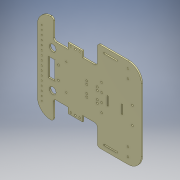
# Autodesk Inventor part: КВ33.035.002 - Платформа 3мм
Saved by Autodesk Inventor 2017 SP1 (Build 210196100, 196)
## iProperties
Part Number: КВ33.035.002 - Платформа 3мм
Material: Типовые
Document SubType Name: Modeling
Designer: sbnnl
Density: 1 g/cm^3
Appearance: Гладкий — пепельный
Author: sbnnl
Autodesk Inventor part; units mm, degrees
ref_plane "YZ Plane" through (0, 0, 0) normal (1, 0, 0) x (0, 1, 0)
ref_plane "XZ Plane" through (0, 0, 0) normal (0, 1, 0) x (-1, 0, 0)
ref_plane "XY Plane" through (0, 0, 0) normal (0, 0, 1) x (1, 0, 0)
sketch "Эскиз1" plane through (0, 0, 0) normal (0, 1, 0) x (-1, 0, 0)
  line L0 (0, 0) -> (93.3924, 0) construction
  line L1 (0, 72) -> (0, 0)
  line L2 (236.5, 0) -> (236.5, 72)
  line L3 (166.5, 57) -> (166.5, 70)
  line L4 (166.5, 70) -> (133.5, 70)
  line L5 (133.5, 70) -> (133.5, 57)
  line L6 (200, 57) -> (166.5, 57)
  line L7 (133.5, 57) -> (100, 57)
  line L8 (170.1825, 65) -> (127.9093, 65) construction
  circle A0 centre (150, 65) radius 2
  circle A1 centre (160, 65) radius 2
  circle A2 centre (140, 65) radius 2
  line L9 (150, 70) -> (150, 80.9563) construction
  line L10 (200, 57) -> (200, 102)
  line L11 (206.5, 102) -> (200, 102)
  line L12 (100, 57) -> (100, 102)
  line L13 (100, 102) -> (30, 102)
  arc A3 (236.5, 72) -> (206.5, 102) centre (206.5, 72) ccw
  arc A4 (30, 102) -> (0, 72) centre (30, 72) ccw
  line L14 (0, -72) -> (0, 0)
  line L15 (236.5, 0) -> (236.5, -72)
  line L16 (166.5, -70) -> (133.5, -70)
  line L17 (133.5, -70) -> (133.5, -57)
  line L18 (200, -57) -> (166.5, -57)
  line L19 (133.5, -57) -> (100, -57)
  line L20 (170.1825, -65) -> (127.9093, -65) construction
  circle A5 centre (150, -65) radius 2
  circle A6 centre (140, -65) radius 2
  line L21 (150, -70) -> (150, -80.9563) construction
  line L22 (200, -57) -> (200, -102)
  line L23 (206.5, -102) -> (200, -102)
  line L24 (100, -57) -> (100, -102)
  line L25 (100, -102) -> (30, -102)
  arc A7 (206.5, -102) -> (236.5, -72) centre (206.5, -72) ccw
  arc A8 (0, -72) -> (30, -102) centre (30, -72) ccw
  line L26 (166.5, -57) -> (166.5, -70)
  circle A9 centre (160, -65) radius 2
  dimension "d0" = 13
  dimension "d1" = 33
  dimension "d2" = 5
  dimension "d3" = 4
  dimension "d4" = 4
  dimension "d5" = 4
  dimension "d6" = 10
  dimension "d7" = 10
  dimension "d8" = 70
  dimension "d9" = 50
  dimension "d11" = 50
  dimension "d12" = 45
  dimension "d13" = 100
  dimension "d14" = 65
  dimension "d15" = 30
  constraints: 54 end point, 21 symmetric about line, 10 centre point, 10 point on line, 8 point on circle, 7 perpendicular, 4 horizontal, 4 tangent, 4 vertical, 2 collinear, 1 equal radius, 1 midpoint, 1 parallel, 5 other
  measures "d0" distance of L3.start L3.end
  measures "d1" distance of L3.end L4.end
  measures "d2" distance between parallel lines of L8 L4
  measures "d3" diameter of A0
  measures "d4" diameter of A1
  measures "d5" diameter of A2
  measures "d6" distance of A1.centre A0.centre
  measures "d7" distance of A2.centre A0.centre
  measures "d8" distance between parallel lines of L2 L3
  measures "d9" distance between parallel lines of L9 L10
  measures "d11" distance between parallel lines of L12 L9
  measures "d12" distance of L7.end L12.end
  measures "d13" distance between parallel lines of L12 L1
  measures "d14" distance between parallel lines of L0 L8
  measures "d15" radius of A3
extrude "Выдавливание1" add sketch "Эскиз1" along normal blind 3
sketch "Эскиз2" plane through (0, 3, 0) normal (0, 1, 0) x (1, 0, 0)
  line L0 (-20, -13.2915) -> (-20, 12.9921) construction
  circle A0 centre (-20, -20) radius 2
  circle A1 centre (-20, 20) radius 2
  point P0 (0, 0)
  dimension "d18" = 4
  dimension "d19" = 20
  dimension "d20" = 40
  dimension "d21" = 20
  constraints: 2 centre point, 2 end point, 2 point on line, 1 equal radius, 1 vertical
  measures "d18" diameter of A1
  measures "d19" distance from line of L0 point (0, 0)
  measures "d20" distance of A1.centre A0.centre
  measures "d21" horizontal distance of point (0, 0) A0.centre
extrude "Выдавливание2" cut sketch "Эскиз2" against normal blind 4
sketch "Эскиз3" plane through (0, 3, 0) normal (0, 1, 0) x (1, 0, 0)
  line L0 (-211.5, -21) -> (-196.5, -21)
  line L1 (-196.5, -21) -> (-196.5, 21)
  line L2 (-196.5, 21) -> (-211.5, 21)
  line L3 (-211.5, 21) -> (-211.5, -21)
  line L4 (-236.5, 72) -> (-236.5, -72) projected
  line L5 (-188.5, -21.5288) -> (-188.5, 22.9768) construction
  circle A0 centre (-188.5, -15) radius 2
  circle A1 centre (-188.5, 15) radius 2
  point P0 (0, 0)
  dimension "d24" = 42
  dimension "d25" = 15
  dimension "d26" = 40
  dimension "d27" = 21
  dimension "d28" = 4
  dimension "d29" = 4
  dimension "d31" = 6
  dimension "d32" = 8
  dimension "d33" = 30
  constraints: 10 end point, 2 centre point, 2 parallel, 2 point on line, 1 horizontal, 1 perpendicular, 1 vertical
  measures "d24" distance of L2.end L0.start
  measures "d25" distance of L1.end L2.end
  measures "d26" distance between parallel lines of L4 L1
  measures "d27" distance from line of point (0, 0) L2
  measures "d28" diameter of A0
  measures "d29" diameter of A1
  measures "d31" distance from line of A1.centre L2
  measures "d32" distance between parallel lines of L1 L5
  measures "d33" distance of A1.centre A0.centre
extrude "Выдавливание3" cut sketch "Эскиз3" against normal blind 4
sketch "Эскиз5" plane through (0, 3, 0) normal (0, 1, 0) x (1, 0, 0)
  line L0 (-134.2143, -16) -> (-95.4487, -16) construction
  circle A0 centre (-100, -16) radius 2
  line L1 (-100, -57) -> (-100, -102) projected
  line L2 (-100, -102) -> (-30, -102) projected
  line L3 (-236.5, -72) -> (-236.5, 72) projected
  line L4 (-236.5, 0) -> (-246.7698, 0) construction
  line L5 (-226.5, -8.1668) -> (-226.5, -72) construction
  circle A1 centre (-226.5, -5) radius 1.5
  circle A2 centre (-226.5, -15) radius 1.5
  circle A3 centre (-226.5, -25) radius 1.5
  circle A4 centre (-226.5, -35) radius 1.5
  circle A5 centre (-226.5, -45) radius 1.5
  circle A6 centre (-226.5, -55) radius 1.5
  circle A7 centre (-226.5, -65) radius 1.5
  circle A8 centre (-226.5, -75) radius 1.5
  circle A9 centre (-226.5, 5) radius 1.5
  circle A10 centre (-226.5, -5) radius 1.5
  circle A11 centre (-226.5, -15) radius 1.5
  circle A12 centre (-226.5, -25) radius 1.5
  circle A13 centre (-226.5, -35) radius 1.5
  circle A14 centre (-226.5, -45) radius 1.5
  circle A15 centre (-226.5, -55) radius 1.5
  circle A16 centre (-226.5, -65) radius 1.5
  circle A17 centre (-226.5, 15) radius 1.5
  circle A18 centre (-226.5, 5) radius 1.5
  circle A19 centre (-226.5, -5) radius 1.5
  circle A20 centre (-226.5, -15) radius 1.5
  circle A21 centre (-226.5, -25) radius 1.5
  circle A22 centre (-226.5, -35) radius 1.5
  circle A23 centre (-226.5, -45) radius 1.5
  circle A24 centre (-226.5, -55) radius 1.5
  circle A25 centre (-226.5, 25) radius 1.5
  circle A26 centre (-226.5, 15) radius 1.5
  circle A27 centre (-226.5, 5) radius 1.5
  circle A28 centre (-226.5, -5) radius 1.5
  circle A29 centre (-226.5, -15) radius 1.5
  circle A30 centre (-226.5, -25) radius 1.5
  circle A31 centre (-226.5, -35) radius 1.5
  circle A32 centre (-226.5, -45) radius 1.5
  circle A33 centre (-226.5, 35) radius 1.5
  circle A34 centre (-226.5, 25) radius 1.5
  circle A35 centre (-226.5, 15) radius 1.5
  circle A36 centre (-226.5, 5) radius 1.5
  circle A37 centre (-226.5, -5) radius 1.5
  circle A38 centre (-226.5, -15) radius 1.5
  circle A39 centre (-226.5, -25) radius 1.5
  circle A40 centre (-226.5, -35) radius 1.5
  circle A41 centre (-226.5, 45) radius 1.5
  circle A42 centre (-226.5, 35) radius 1.5
  circle A43 centre (-226.5, 25) radius 1.5
  circle A44 centre (-226.5, 15) radius 1.5
  circle A45 centre (-226.5, 5) radius 1.5
  circle A46 centre (-226.5, -5) radius 1.5
  circle A47 centre (-226.5, -15) radius 1.5
  circle A48 centre (-226.5, -25) radius 1.5
  circle A49 centre (-226.5, 55) radius 1.5
  circle A50 centre (-226.5, 45) radius 1.5
  circle A51 centre (-226.5, 35) radius 1.5
  circle A52 centre (-226.5, 25) radius 1.5
  circle A53 centre (-226.5, 15) radius 1.5
  circle A54 centre (-226.5, 5) radius 1.5
  circle A55 centre (-226.5, -5) radius 1.5
  circle A56 centre (-226.5, -15) radius 1.5
  circle A57 centre (-226.5, 65) radius 1.5
  circle A58 centre (-226.5, 55) radius 1.5
  circle A59 centre (-226.5, 45) radius 1.5
  circle A60 centre (-226.5, 35) radius 1.5
  circle A61 centre (-226.5, 25) radius 1.5
  circle A62 centre (-226.5, 15) radius 1.5
  circle A63 centre (-226.5, 5) radius 1.5
  circle A64 centre (-226.5, -5) radius 1.5
  circle A65 centre (-226.5, 75) radius 1.5
  circle A66 centre (-226.5, 65) radius 1.5
  circle A67 centre (-226.5, 55) radius 1.5
  circle A68 centre (-226.5, 45) radius 1.5
  circle A69 centre (-226.5, 35) radius 1.5
  circle A70 centre (-226.5, 25) radius 1.5
  circle A71 centre (-226.5, 15) radius 1.5
  circle A72 centre (-226.5, 5) radius 1.5
  line L6 (-78, -10) -> (-75, -10)
  line L7 (-75, -10) -> (-75, 10)
  line L8 (-75, 10) -> (-78, 10)
  line L9 (-78, 10) -> (-78, -10)
  line L10 (-133.5, -70) -> (-133.5, -57) projected
  line L11 (-45, -10) -> (-42, -10)
  line L12 (-42, -10) -> (-42, 10)
  line L13 (-42, 10) -> (-45, 10)
  line L14 (-45, 10) -> (-45, -10)
  line L15 (-100, -16) -> (-100, 38.9096) construction
  circle A73 centre (-100, 16) radius 2
  circle A74 centre (-100, 9) radius 2
  circle A75 centre (-100, -9) radius 2
  circle A76 centre (-124, -16) radius 2
  circle A77 centre (-124, -9) radius 2
  circle A78 centre (-124, 9) radius 2
  circle A79 centre (-124, 16) radius 2
  line L16 (-100, 16) -> (-119.6213, 16) construction
  line L17 (-170.5, 43.1181) -> (-170.5, -35.1229) construction
  circle A80 centre (-170.5, 30.25) radius 1.5
  circle A81 centre (-170.5, -30.25) radius 1.5
  point P0 (0, 0)
  dimension "d38" = 4
  dimension "d52" = 3
  dimension "d53" = 10
  dimension "d54" = 5
  dimension "d57" = 10
  dimension "d60" = 10
  dimension "d63" = 20
  dimension "d64" = 3
  dimension "d65" = 10
  dimension "d68" = 33
  dimension "d105" = 32
  dimension "d106" = 25
  dimension "d114" = 25
  dimension "d117" = 24
  dimension "d122" = 42
  dimension "d123" = 22
  dimension "d124" = 16
  dimension "d126" = 3
  dimension "d127" = 3
  dimension "d128" = 60.5
  dimension "d129" = 30.25
  dimension "d130" = 66
  constraints: 82 centre point, 28 end point, 7 point on line, 5 horizontal, 5 vertical, 3 equal radius, 2 parallel, 1 midpoint, 1 perpendicular, 159 other
  measures "d38" diameter of A0
  measures "d52" diameter of A1
  measures "d53" distance between parallel lines of L3 L5
  measures "d54" distance from line of A1.centre L4
  measures "d57" distance of A1.centre A2.centre
  measures "d60" distance of A1.centre A9.centre
  measures "d63" distance of L8.end L6.start
  measures "d64" distance of L7.end L8.end
  measures "d65" distance between parallel lines of L4 L8
  measures "d68" distance of L6.end L11.end
  measures "d105" distance of L16.start L15.start
  measures "d106" distance of A74.centre L15.start
  measures "d114" distance of A75.centre L16.start
  measures "d117" distance of L15.start A76.centre
  measures "d122" distance from line of point (0, 0) L12
  measures "d123" distance between parallel lines of L15 L9
  measures "d124" distance between parallel lines of L4 L16
  measures "d126" diameter of A80
  measures "d127" diameter of A81
  measures "d128" distance of A81.centre A80.centre
  measures "d129" distance from line of L4 A81.centre
  measures "d130" distance between parallel lines of L17 L3
extrude "Выдавливание5" cut sketch "Эскиз5" against normal blind 4
sketch "Эскиз6" plane through (0, 3, 0) normal (0, 1, 0) x (1, 0, 0)
  line L0 (-201.5, -38.8438) -> (-201.5, 45.9723) construction
  circle A0 centre (-201.5, -42) radius 7.5
  circle A1 centre (-201.5, 42) radius 7.5
  line L1 (-200, -57) -> (-166.5, -57) projected
  line L2 (-166.5, 57) -> (-200, 57) projected
  line L3 (-236.5, -72) -> (-236.5, 72) projected
  point P0 (0, 0)
  dimension "d75" = 15
  dimension "d76" = 15
  dimension "d77" = 15
  dimension "d78" = 15
  dimension "d79" = 35
  constraints: 2 centre point, 2 end point, 2 point on line, 1 vertical
  measures "d75" diameter of A0
  measures "d76" diameter of A1
  measures "d77" distance from line of A0.centre L1
  measures "d78" distance from line of A1.centre L2
  measures "d79" distance between parallel lines of L3 L0
extrude "Выдавливание6" cut sketch "Эскиз6" against normal blind 10
sketch "Эскиз7" plane through (0, 3, 0) normal (0, 1, 0) x (1, 0, 0)
  line L0 (-90, -53.2705) -> (-90, -1.5372) construction
  circle A0 centre (-90, -30) radius 2
  line L1 (-90, -33.2705) -> (-90, 18.4628) construction
  circle A1 centre (-90, -10) radius 2
  line L2 (-90, -13.2705) -> (-90, 38.4628) construction
  circle A2 centre (-90, 10) radius 2
  line L3 (-90, 6.7295) -> (-90, 58.4628) construction
  circle A3 centre (-90, 30) radius 2
  point P0 (0, 0)
  dimension "d82" = 4
  dimension "d83" = 30
  dimension "d84" = 90
  dimension "d87" = 20
  constraints: 8 end point, 4 centre point, 4 point on line, 2 vertical, 1 collinear, 14 other
  measures "d82" diameter of A0
  measures "d83" vertical distance of A0.centre point (0, 0)
  measures "d84" distance from line of point (0, 0) L0
  measures "d87" distance of L0.start L1.start
extrude "Выдавливание7" cut sketch "Эскиз7" against normal blind 10
sketch "Эскиз8" plane through (0, 3, 0) normal (0, 1, 0) x (1, 0, 0)
  line L0 (-85, 89) -> (-55, 89)
  line L1 (-55, 89) -> (-55, 92)
  line L2 (-55, 92) -> (-85, 92)
  line L3 (-85, 92) -> (-85, 89)
  line L4 (-30, 102) -> (-100, 102) projected
  line L5 (-100, 102) -> (-100, 57) projected
  line L6 (-30, 60.9127) -> (-30, 96.4392) construction
  circle A0 centre (-30, 67) radius 2
  circle A1 centre (-30, 87) radius 2
  line L7 (0, -72) -> (0, 72) projected
  line L8 (0, 0) -> (41.7371, 0) construction
  line L9 (-85, -89) -> (-55, -89)
  line L10 (-55, -89) -> (-55, -92)
  line L11 (-55, -92) -> (-85, -92)
  line L12 (-85, -92) -> (-85, -89)
  line L13 (-100, -102) -> (-100, -57)
  line L14 (-30, -60.9127) -> (-30, -96.4392) construction
  circle A2 centre (-30, -67) radius 2
  circle A3 centre (-30, -87) radius 2
  dimension "d94" = 3
  dimension "d95" = 10
  dimension "d96" = 15
  dimension "d97" = 30
  dimension "d98" = 4
  dimension "d99" = 4
  dimension "d100" = 30
  dimension "d101" = 15
  dimension "d102" = 20
  constraints: 24 end point, 10 symmetric about line, 4 centre point, 4 point on line, 2 horizontal, 2 parallel, 1 perpendicular, 1 vertical, 2 other
  measures "d94" distance of L2.end L0.start
  measures "d95" distance between parallel lines of L4 L2
  measures "d96" distance between parallel lines of L3 L5
  measures "d97" distance of L1.end L2.end
  measures "d98" diameter of A0
  measures "d99" diameter of A1
  measures "d100" distance between parallel lines of L6 L7
  measures "d101" distance from line of L4 A1.centre
  measures "d102" distance of A0.centre A1.centre
extrude "Выдавливание8" cut sketch "Эскиз8" against normal blind 10
fillet "Сопряжение1" radius 6 8 edges at (-200, 1.5, 57) (-100, 1.5, 57) (-100, 1.5, -57) (-200, 1.5, -57) (-100, 1.5, 102) (-200, 1.5, 102) (-100, 1.5, -102) (-200, 1.5, -102)
